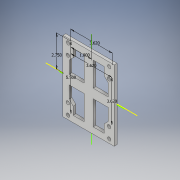
# Autodesk Inventor part: MotorAdapter
Saved by Autodesk Inventor 2018 (Build 220112000, 112)
## iProperties
Created: 2017-05-04
Part Number: MotorAdapter
Material: Generic
Document SubType Name: Modeling
Designer: boss
Density: 1 g/cm^3
Appearance: Default
Author: boss
Autodesk Inventor part; units mm, degrees
ref_plane "YZ Plane" through (0, 0, 0) normal (1, 0, 0) x (0, 1, 0)
ref_plane "XZ Plane" through (0, 0, 0) normal (0, 1, 0) x (-1, 0, 0)
ref_plane "XY Plane" through (0, 0, 0) normal (0, 0, 1) x (1, 0, 0)
sketch "Sketch1" plane through (0, 0, 0) normal (0, 0, 1) x (-1, 0, 0)
  line L0 (-57.15, 78.74) -> (57.15, 78.74)
  line L1 (57.15, 78.74) -> (57.15, -78.74)
  line L2 (57.15, -78.74) -> (-57.15, -78.74)
  line L3 (-57.15, -78.74) -> (-57.15, 78.74)
  line L4 (-57.15, 78.74) -> (57.15, -78.74) construction
  line L5 (57.15, 78.74) -> (-57.15, -78.74) construction
  point P0 (0, 0)
  dimension "d0" = 114.3
  dimension "d1" = 157.48
  constraints: 12 end point, 2 midpoint, 2 parallel, 1 horizontal, 1 perpendicular
  measures "d0" distance of L1.end L2.end
  measures "d1" distance of L0.end L1.end
extrude "Extrusion1" add sketch "Sketch1" along normal blind 6.35
sketch "Sketch2" plane through (0, 0, 0) normal (0, 0, 1) x (1, 0, 0)
  line L0 (0, 106.68) -> (0, -106.68)
  line L1 (72.898, -1.6229) -> (-72.898, -1.6229)
  line L2 (0, -106.68) -> (0, 106.68)
  line L3 (-102.0572, 0) -> (102.0572, 0) projected
  point P0 (45.72, 45.72)
  point P1 (-46.228, 45.72)
  point P2 (45.72, -46.228)
  point P3 (-46.228, -46.228)
  point P4 (-45.72, 69.85)
  point P5 (-45.72, -69.85)
  point P6 (46.228, 69.85)
  point P7 (46.228, -69.85)
  dimension "d18" = 91.948
  dimension "d21" = 91.948
  dimension "d25" = 45.72
  dimension "d28" = 139.7
  dimension "d31" = 91.948
  dimension "d34" = 69.85
  constraints: 6 end point, 2 horizontal, 2 vertical, 6 other
  measures "d18" distance of point (45.72, 45.72) point (-46.228, 45.72)
  measures "d21" distance of point (45.72, 45.72) point (45.72, -46.228)
  measures "d25" distance from line of point (-45.72, 69.85) L0
  measures "d28" distance of point (-45.72, 69.85) point (-45.72, -69.85)
  measures "d31" distance of point (-45.72, 69.85) point (46.228, 69.85)
  measures "d34" distance from line of point (-45.72, 69.85) L3
hole "Hole1" at (45.72, 45.72, 0) at (-46.228, 45.72, 0) at (-46.228, -46.228, 0) at (45.72, -46.228, 0) at (-45.72, 69.85, 0) at (46.228, 69.85, 0) at (-45.72, -69.85, 0) at (46.228, -69.85, 0) direction (0, 0, 1) diameter 7.62 end through all
sketch "Sketch6" plane through (0, 0, 6.35) normal (0, 0, 1) x (1, 0, 0)
  line L0 (-10.16, 10.16) -> (-43.434, 10.16)
  line L1 (-43.434, 10.16) -> (-43.434, 37.846)
  line L2 (-43.434, 37.846) -> (-10.16, 37.846)
  line L3 (-10.16, 37.846) -> (-10.16, 10.16)
  line L4 (-80.01, 0) -> (80.01, 0) projected
  line L5 (0, -110.236) -> (0, 110.236) projected
  line L6 (-43.434, 37.846) -> (-11.5677, 37.846) construction
  line L7 (-43.434, 37.846) -> (-7.62, 37.846) construction
  line L8 (-43.434, 37.846) -> (-34.4537, 46.8263)
  line L9 (-43.434, 37.846) -> (-30.734, 37.846) construction
  line L10 (-34.4537, 46.8263) -> (-10.16, 46.8263)
  line L11 (-10.16, 46.8263) -> (-10.16, 64.6111)
  line L12 (-10.16, 64.6111) -> (-34.4537, 64.6111)
  line L13 (-34.4537, 64.6111) -> (-34.4537, 46.8263)
  line L14 (-10.16, 46.8263) -> (-10.16, 37.846)
  line L15 (10.16, 10.16) -> (43.434, 10.16)
  line L16 (43.434, 10.16) -> (43.434, 37.846)
  line L17 (43.434, 37.846) -> (10.16, 37.846)
  line L18 (10.16, 37.846) -> (10.16, 10.16)
  line L19 (43.434, 37.846) -> (11.5677, 37.846) construction
  line L20 (43.434, 37.846) -> (7.62, 37.846) construction
  line L21 (43.434, 37.846) -> (34.4537, 46.8263)
  line L22 (43.434, 37.846) -> (30.734, 37.846) construction
  line L23 (34.4537, 46.8263) -> (10.16, 46.8263)
  line L24 (10.16, 46.8263) -> (10.16, 64.6111)
  line L25 (10.16, 64.6111) -> (34.4537, 64.6111)
  line L26 (34.4537, 64.6111) -> (34.4537, 46.8263)
  line L27 (10.16, 46.8263) -> (10.16, 37.846)
  line L28 (-10.16, -10.16) -> (-43.434, -10.16)
  line L29 (-43.434, -10.16) -> (-43.434, -37.846)
  line L30 (-43.434, -37.846) -> (-10.16, -37.846)
  line L31 (-10.16, -37.846) -> (-10.16, -10.16)
  line L32 (-43.434, -37.846) -> (-11.5677, -37.846) construction
  line L33 (-43.434, -37.846) -> (-7.62, -37.846) construction
  line L34 (-43.434, -37.846) -> (-34.4537, -46.8263)
  line L35 (-43.434, -37.846) -> (-30.734, -37.846) construction
  line L36 (-34.4537, -46.8263) -> (-10.16, -46.8263)
  line L37 (-10.16, -46.8263) -> (-10.16, -64.6111)
  line L38 (-10.16, -64.6111) -> (-34.4537, -64.6111)
  line L39 (-34.4537, -64.6111) -> (-34.4537, -46.8263)
  line L40 (-10.16, -46.8263) -> (-10.16, -37.846)
  line L41 (10.16, -10.16) -> (43.434, -10.16)
  line L42 (43.434, -10.16) -> (43.434, -37.846)
  line L43 (10.16, -37.846) -> (10.16, -10.16)
  line L44 (43.434, -37.846) -> (10.16, -37.846)
  line L45 (43.434, -37.846) -> (11.5677, -37.846) construction
  line L46 (43.434, -37.846) -> (30.734, -37.846) construction
  line L47 (10.16, -46.8263) -> (10.16, -37.846)
  line L48 (34.4537, -46.8263) -> (10.16, -46.8263)
  line L49 (43.434, -37.846) -> (34.4537, -46.8263)
  line L50 (10.16, -46.8263) -> (10.16, -64.6111)
  line L51 (10.16, -64.6111) -> (34.4537, -64.6111)
  line L52 (34.4537, -64.6111) -> (34.4537, -46.8263)
  line L53 (43.434, -37.846) -> (7.62, -37.846) construction
  point P0 (0, 0)
  dimension "d41" = 10.16
  dimension "d42" = 10.16
  dimension "d43" = 43.434
  dimension "d44" = 37.846
  dimension "d54" = 12.7
  dimension "d55" = 45
  constraints: 104 end point, 33 symmetric about line, 5 horizontal, 4 parallel, 2 perpendicular, 1 equal length, 1 vertical
  measures "d41" distance between parallel lines of L4 L0
  measures "d42" distance between parallel lines of L5 L3
  measures "d43" distance between parallel lines of L5 L1
  measures "d44" distance between parallel lines of L4 L2
  measures "d54" distance of L1.end L8.end
  measures "d55" angle of L9 L8
extrude "Extrusion3" cut sketch "Sketch6" against normal blind 25.4
equation "\"d12\" = d18"
body "Solid1"
